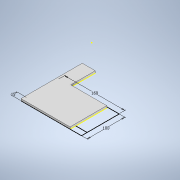
# Autodesk Inventor part: board_R
Saved by Autodesk Inventor 2020 (Build 240168000, 168)
## iProperties
Created: 2022-07-25
Part Number: board_R
Material: 일반
Document SubType Name: Modeling
Designer: SeungJin
Density: 1 g/cm^3
Appearance: 기본값
Author: SeungJin
Autodesk Inventor part; units mm, degrees
ref_plane "YZ Plane" through (0, 0, 0) normal (1, 0, 0) x (0, 1, 0)
ref_plane "XZ Plane" through (0, 0, 0) normal (0, 1, 0) x (-1, 0, 0)
ref_plane "XY Plane" through (0, 0, 0) normal (0, 0, 1) x (1, 0, 0)
ref_plane "작업 평면1" through (150.5, 0, 75) normal (0, 1, 0) x (1, 0, 0)
sketch "스케치1" plane through (150.5, 0, 75) normal (0, 1, 0) x (1, 0, 0)
  line L0 (75, -152.5) -> (-110.5, -152.5)
  line L1 (75, 0) -> (75, -152.5)
  line L2 (0, 0) -> (75, 0)
  line L3 (0, 10) -> (0, 0)
  line L4 (-110.5, 10) -> (0, 10)
  line L5 (-110.5, 10) -> (0, 10)
  line L6 (-110.5, 10) -> (-110.5, -152.5)
  line L7 (75, 10) -> (-76, 10)
  line L8 (-76, 10) -> (-76, -55)
  line L9 (-76, -55) -> (75, -55)
  line L10 (75, -55) -> (75, 10)
  line L11 (19.5, -55) -> (19.5, -152.5)
  point P0 (-150.5, 75)
  point P1 (-76, 10)
  dimension "d19" = 151
  dimension "d20" = 65
  dimension "d21" = 130
  dimension "d24" = 185.5
  constraints: 24 end point, 3 perpendicular, 2 parallel, 2 point on line, 1 horizontal, 7 other
  measures "d19" distance of L9.end L8.end
  measures "d20" distance of L8.end L7.end
  measures "d21" distance between parallel lines of L6 L11
  measures "d24" distance of L0.start L0.end
extrude "돌출1" add sketch "스케치1" along normal blind 5 contours L0 L6 L4 L8 L9 L11
sketch "스케치2" plane through (150.5, 0, 75) normal (0, -1, 0) x (1, 0, 0)
  line L0 (-110.5, 152.5) -> (19.5, 152.5) projected
  line L1 (-110.5, -10) -> (-110.5, 152.5) projected
  line L2 (-76, -10) -> (-110.5, -10) projected
  line L3 (-76, 55) -> (-76, -10) projected
  line L4 (19.5, 55) -> (-76, 55) projected
  line L5 (19.5, 152.5) -> (19.5, 55) projected
  line L6 (-110.5, 152.5) -> (49.5, 152.5)
  line L7 (49.5, 152.5) -> (49.5, 52.5)
  line L8 (49.5, 52.5) -> (-110.5, 52.5)
  line L9 (-110.5, 52.5) -> (-110.5, 152.5)
  line L10 (-110.5, 137.5) -> (49.5, 137.5)
  point P0 (-150.5, -75)
  dimension "d22" = 160
  dimension "d23" = 100
  dimension "d25" = 15
  constraints: 10 end point, 2 parallel, 2 perpendicular, 2 point on line, 1 horizontal
  measures "d22" distance of L7.end L8.end
  measures "d23" distance of L6.end L7.end
  measures "d25" distance between parallel lines of L6 L10
